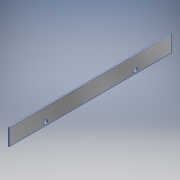
# Autodesk Inventor part: Bumper Plate
Saved by Autodesk Inventor 2019.4 (Build 234330000, 330)
## iProperties
Created: 2019-10-20
Part Number: Bumper Plate
Material: Aluminum 6061
Document SubType Name: Modeling
Designer: admin
Density: 2.7 g/cm^3
Appearance: Aluminum - Flat
Mass: 1233.5 g
Surface Area: 1935.72 cm^2
Volume: 456.852 cm^3
Author: admin
Autodesk Inventor part; units mm, degrees
ref_plane "YZ Plane" through (0, 0, 0) normal (1, 0, 0) x (0, 1, 0)
ref_plane "XZ Plane" through (0, 0, 0) normal (0, 1, 0) x (-1, 0, 0)
ref_plane "XY Plane" through (0, 0, 0) normal (0, 0, 1) x (1, 0, 0)
sketch "Sketch1" plane through (0, 0, 0) normal (1, 0, 0) x (0, 1, 0)
  line L0 (-50, 489.5) -> (50, 489.5)
  line L1 (50, 489.5) -> (50, -489.5)
  line L2 (50, -489.5) -> (-50, -489.5)
  line L3 (-50, -489.5) -> (-50, 489.5)
  line L4 (-50, 489.5) -> (50, -489.5) construction
  line L5 (50, 489.5) -> (-50, -489.5) construction
  point P0 (0, 0)
  dimension "d0" = 979
  dimension "d1" = 100
  constraints: 12 end point, 2 midpoint, 2 parallel, 1 horizontal, 1 perpendicular
  measures "d0" distance of L0.end L1.end
  measures "d1" distance of L0.start L0.end
extrude "Extrusion1" add sketch "Sketch1" along normal blind 5
sketch "Sketch2" plane through (5, 0, 0) normal (1, 0, 0) x (0, 0, -1)
  circle A0 centre (-270.411, -31.452) radius 12.25
  line L0 (-489.5, -50) -> (489.5, -50) projected
  line L1 (-489.5, 50) -> (-489.5, -50) projected
  circle A1 centre (270.589, -31.452) radius 12.25
  line L2 (489.5, -50) -> (489.5, 50) projected
  point P0 (0, 0)
  dimension "d4" = 24.5
  dimension "d5" = 18.548
  dimension "d8" = 219.089
  dimension "d18" = 218.911
  dimension "d19" = 24.5
  dimension "d20" = 18.548
  constraints: 2 centre point
  measures "d4" diameter of A0
  measures "d5" distance from line of L0 A0.centre
  measures "d8" distance from line of L1 A0.centre
  measures "d18" distance from line of L2 A1.centre
  measures "d19" diameter of A1
  measures "d20" distance from line of L0 A1.centre
extrude "Extrusion2" cut sketch "Sketch2" against normal through all
equation "\"d20\" = d5"
body "Solid1"
